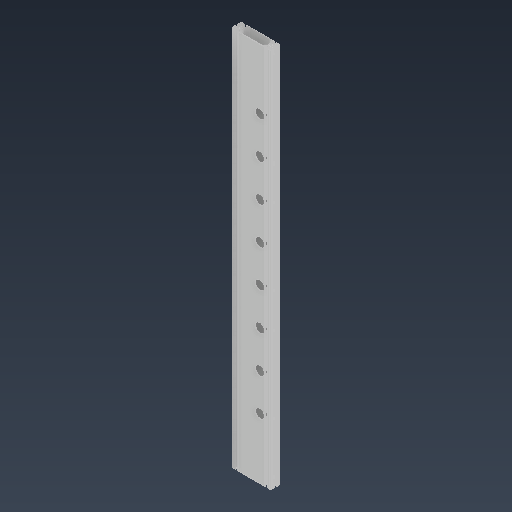
# Autodesk Inventor part: tallBeamLong
Saved by Autodesk Inventor 2021.4 (Build 254397000, 397)
## iProperties
Created: 2021-11-23
Part Number: tallBeamLong
Material: Generic
Document SubType Name: Modeling
Designer: jo_ki
Density: 1 g/cm^3
Appearance: Aluminum - Dark
Author: jo_ki
Autodesk Inventor part; units mm, degrees
ref_plane "YZ Plane" through (0, 0, 0) normal (1, 0, 0) x (0, 1, 0)
ref_plane "XZ Plane" through (0, 0, 0) normal (0, 1, 0) x (-1, 0, 0)
ref_plane "XY Plane" through (0, 0, 0) normal (0, 0, 1) x (1, 0, 0)
derived "Item_Profil_Hoch.ipt"
sketch "Skizze4" plane through (-54.5, 30, -20) normal (0, 1, 0) x (1, 0, 0)
  circle A0 centre (-5.5, -20) radius 3.4
  point P0 (54.5, -20)
sketch "Sketch9" plane through (0, 0, 0) normal (0, 1, 0) x (-1, 0, 0)
  line L0 (-78.3725, 16) -> (-78.3725, 12.3)
  arc A0 (-78.3725, 12.3) -> (-77.8725, 11.8) centre (-77.8725, 12.3) ccw
  line L1 (-77.8725, 11.8) -> (-72.4725, 11.8)
  arc A1 (-72.4725, 11.8) -> (-71.9725, 12.3) centre (-72.4725, 12.3) ccw
  line L2 (-71.9725, 12.3) -> (-71.9725, 17.7)
  arc A2 (-71.9725, 17.7) -> (-72.4725, 18.2) centre (-72.4725, 17.7) ccw
  line L3 (-72.4725, 18.2) -> (-76.1725, 18.2)
  arc A3 (-76.1725, 18.2) -> (-78.3725, 16) centre (-76.1725, 16) ccw
  line L4 (78.3725, -16) -> (78.3725, -12.3)
  arc A4 (78.3725, -12.3) -> (77.8725, -11.8) centre (77.8725, -12.3) ccw
  line L5 (77.8725, -11.8) -> (72.4725, -11.8)
  arc A5 (72.4725, -11.8) -> (71.9725, -12.3) centre (72.4725, -12.3) ccw
  line L6 (71.9725, -12.3) -> (71.9725, -17.7)
  arc A6 (71.9725, -17.7) -> (72.4725, -18.2) centre (72.4725, -17.7) ccw
  line L7 (72.4725, -18.2) -> (76.1725, -18.2)
  arc A7 (76.1725, -18.2) -> (78.3725, -16) centre (76.1725, -16) ccw
  line L8 (-76, -18.3725) -> (-72.3, -18.3725)
  arc A8 (-72.3, -18.3725) -> (-71.8, -17.8725) centre (-72.3, -17.8725) ccw
  line L9 (-71.8, -17.8725) -> (-71.8, -12.4725)
  arc A9 (-71.8, -12.4725) -> (-72.3, -11.9725) centre (-72.3, -12.4725) ccw
  line L10 (-72.3, -11.9725) -> (-77.7, -11.9725)
  arc A10 (-77.7, -11.9725) -> (-78.2, -12.4725) centre (-77.7, -12.4725) ccw
  line L11 (-78.2, -12.4725) -> (-78.2, -16.1725)
  arc A11 (-78.2, -16.1725) -> (-76, -18.3725) centre (-76, -16.1725) ccw
  line L12 (76, 18.3725) -> (72.3, 18.3725)
  arc A12 (72.3, 18.3725) -> (71.8, 17.8725) centre (72.3, 17.8725) ccw
  line L13 (71.8, 17.8725) -> (71.8, 12.4725)
  arc A13 (71.8, 12.4725) -> (72.3, 11.9725) centre (72.3, 12.4725) ccw
  line L14 (72.3, 11.9725) -> (77.7, 11.9725)
  arc A14 (77.7, 11.9725) -> (78.2, 12.4725) centre (77.7, 12.4725) ccw
  line L15 (78.2, 12.4725) -> (78.2, 16.1725)
  arc A15 (78.2, 16.1725) -> (76, 18.3725) centre (76, 16.1725) ccw
  circle A16 centre (60, 0) radius 3.4
  circle A17 centre (-60, 0) radius 3.4
  arc A18 (80, -5.5) -> (78.5, -4) centre (78.5, -5.5) ccw
  line L16 (80, -16) -> (80, -5.5)
  arc A19 (76, -20) -> (80, -16) centre (76, -16) ccw
  line L17 (65.5, -20) -> (76, -20)
  arc A20 (64, -18.5) -> (65.5, -20) centre (65.5, -18.5) ccw
  line L18 (64, -18.5) -> (64, -16.5)
  arc A21 (65, -15.5) -> (64, -16.5) centre (65, -16.5) ccw
  line L19 (65, -15.5) -> (66.5, -15.5)
  arc A22 (67, -16) -> (66.5, -15.5) centre (66.5, -16) ccw
  line L20 (67, -16) -> (67, -17.55)
  arc A23 (67, -17.55) -> (67.45, -18) centre (67.45, -17.55) ccw
  line L21 (67.45, -18) -> (67.5, -18)
  arc A24 (67.5, -18) -> (70, -15.5) centre (67.5, -15.5) ccw
  line L22 (70, -15.5) -> (70, -14.1924)
  arc A25 (70, -14.1924) -> (68.5355, -10.6569) centre (65, -14.1924) ccw
  line L23 (68.5355, -10.6569) -> (67.0931, -9.2145)
  arc A26 (67.0931, -9.2145) -> (63.5576, -7.75) centre (63.5576, -12.75) ccw
  line L24 (63.5576, -7.75) -> (56.4424, -7.75)
  arc A27 (56.4424, -7.75) -> (52.9069, -9.2145) centre (56.4424, -12.75) ccw
  line L25 (52.9069, -9.2145) -> (51.4645, -10.6569)
  arc A28 (51.4645, -10.6569) -> (50, -14.1924) centre (55, -14.1924) ccw
  line L26 (50, -14.1924) -> (50, -15.5)
  arc A29 (50, -15.5) -> (52.5, -18) centre (52.5, -15.5) ccw
  line L27 (52.5, -18) -> (52.55, -18)
  arc A30 (52.55, -18) -> (53, -17.55) centre (52.55, -17.55) ccw
  line L28 (53, -17.55) -> (53, -16)
  arc A31 (53.5, -15.5) -> (53, -16) centre (53.5, -16) ccw
  line L29 (53.5, -15.5) -> (55, -15.5)
  arc A32 (56, -16.5) -> (55, -15.5) centre (55, -16.5) ccw
  line L30 (56, -16.5) -> (56, -18.5)
  arc A33 (54.5, -20) -> (56, -18.5) centre (54.5, -18.5) ccw
  line L31 (-54.5, -20) -> (54.5, -20)
  arc A34 (-56, -18.5) -> (-54.5, -20) centre (-54.5, -18.5) ccw
  line L32 (-56, -18.5) -> (-56, -16.5)
  arc A35 (-55, -15.5) -> (-56, -16.5) centre (-55, -16.5) ccw
  line L33 (-55, -15.5) -> (-53.5, -15.5)
  arc A36 (-53, -16) -> (-53.5, -15.5) centre (-53.5, -16) ccw
  line L34 (-53, -16) -> (-53, -17.55)
  arc A37 (-53, -17.55) -> (-52.55, -18) centre (-52.55, -17.55) ccw
  line L35 (-52.55, -18) -> (-52.5, -18)
  arc A38 (-52.5, -18) -> (-50, -15.5) centre (-52.5, -15.5) ccw
  line L36 (-50, -15.5) -> (-50, -14.1924)
  arc A39 (-50, -14.1924) -> (-51.4645, -10.6569) centre (-55, -14.1924) ccw
  line L37 (-51.4645, -10.6569) -> (-52.9069, -9.2145)
  arc A40 (-52.9069, -9.2145) -> (-56.4424, -7.75) centre (-56.4424, -12.75) ccw
  line L38 (-56.4424, -7.75) -> (-63.5576, -7.75)
  arc A41 (-63.5576, -7.75) -> (-67.0931, -9.2145) centre (-63.5576, -12.75) ccw
  line L39 (-67.0931, -9.2145) -> (-68.5355, -10.6569)
  arc A42 (-68.5355, -10.6569) -> (-70, -14.1924) centre (-65, -14.1924) ccw
  line L40 (-70, -14.1924) -> (-70, -15.5)
  arc A43 (-70, -15.5) -> (-67.5, -18) centre (-67.5, -15.5) ccw
  line L41 (-67.5, -18) -> (-67.45, -18)
  arc A44 (-67.45, -18) -> (-67, -17.55) centre (-67.45, -17.55) ccw
  line L42 (-67, -17.55) -> (-67, -16)
  arc A45 (-66.5, -15.5) -> (-67, -16) centre (-66.5, -16) ccw
  line L43 (-66.5, -15.5) -> (-65, -15.5)
  arc A46 (-64, -16.5) -> (-65, -15.5) centre (-65, -16.5) ccw
  line L44 (-64, -16.5) -> (-64, -18.5)
  arc A47 (-65.5, -20) -> (-64, -18.5) centre (-65.5, -18.5) ccw
  line L45 (-76, -20) -> (-65.5, -20)
  arc A48 (-80, -16) -> (-76, -20) centre (-76, -16) ccw
  line L46 (-80, -5.5) -> (-80, -16)
  arc A49 (-78.5, -4) -> (-80, -5.5) centre (-78.5, -5.5) ccw
  line L47 (-78.5, -4) -> (-76.5, -4)
  arc A50 (-75.5, -5) -> (-76.5, -4) centre (-76.5, -5) ccw
  line L48 (-75.5, -5) -> (-75.5, -6.5)
  arc A51 (-76, -7) -> (-75.5, -6.5) centre (-76, -6.5) ccw
  line L49 (-76, -7) -> (-77.55, -7)
  arc A52 (-77.55, -7) -> (-78, -7.45) centre (-77.55, -7.45) ccw
  line L50 (-78, -7.45) -> (-78, -7.5)
  arc A53 (-78, -7.5) -> (-75.5, -10) centre (-75.5, -7.5) ccw
  line L51 (-75.5, -10) -> (-74.1924, -10)
  arc A54 (-74.1924, -10) -> (-70.6569, -8.5355) centre (-74.1924, -5) ccw
  line L52 (-70.6569, -8.5355) -> (-69.2145, -7.0931)
  arc A55 (-69.2145, -7.0931) -> (-67.75, -3.5576) centre (-72.75, -3.5576) ccw
  line L53 (-67.75, -3.5576) -> (-67.75, 3.5576)
  arc A56 (-67.75, 3.5576) -> (-69.2145, 7.0931) centre (-72.75, 3.5576) ccw
  line L54 (-69.2145, 7.0931) -> (-70.6569, 8.5355)
  arc A57 (-70.6569, 8.5355) -> (-74.1924, 10) centre (-74.1924, 5) ccw
  line L55 (-74.1924, 10) -> (-75.5, 10)
  arc A58 (-75.5, 10) -> (-78, 7.5) centre (-75.5, 7.5) ccw
  line L56 (-78, 7.5) -> (-78, 7.45)
  arc A59 (-78, 7.45) -> (-77.55, 7) centre (-77.55, 7.45) ccw
  line L57 (-77.55, 7) -> (-76, 7)
  arc A60 (-75.5, 6.5) -> (-76, 7) centre (-76, 6.5) ccw
  line L58 (-75.5, 6.5) -> (-75.5, 5)
  arc A61 (-76.5, 4) -> (-75.5, 5) centre (-76.5, 5) ccw
  line L59 (-76.5, 4) -> (-78.5, 4)
  arc A62 (-80, 5.5) -> (-78.5, 4) centre (-78.5, 5.5) ccw
  line L60 (-80, 16) -> (-80, 5.5)
  arc A63 (-76, 20) -> (-80, 16) centre (-76, 16) ccw
  line L61 (-65.5, 20) -> (-76, 20)
  arc A64 (-64, 18.5) -> (-65.5, 20) centre (-65.5, 18.5) ccw
  line L62 (-64, 18.5) -> (-64, 16.5)
  arc A65 (-65, 15.5) -> (-64, 16.5) centre (-65, 16.5) ccw
  line L63 (-65, 15.5) -> (-66.5, 15.5)
  arc A66 (-67, 16) -> (-66.5, 15.5) centre (-66.5, 16) ccw
  line L64 (-67, 16) -> (-67, 17.55)
  arc A67 (-67, 17.55) -> (-67.45, 18) centre (-67.45, 17.55) ccw
  line L65 (-67.45, 18) -> (-67.5, 18)
  arc A68 (-67.5, 18) -> (-70, 15.5) centre (-67.5, 15.5) ccw
  line L66 (-70, 15.5) -> (-70, 14.1924)
  arc A69 (-70, 14.1924) -> (-68.5355, 10.6569) centre (-65, 14.1924) ccw
  line L67 (-68.5355, 10.6569) -> (-67.0931, 9.2145)
  arc A70 (-67.0931, 9.2145) -> (-63.5576, 7.75) centre (-63.5576, 12.75) ccw
  line L68 (-63.5576, 7.75) -> (-56.4424, 7.75)
  arc A71 (-56.4424, 7.75) -> (-52.9069, 9.2145) centre (-56.4424, 12.75) ccw
  line L69 (-52.9069, 9.2145) -> (-51.4645, 10.6569)
  arc A72 (-51.4645, 10.6569) -> (-50, 14.1924) centre (-55, 14.1924) ccw
  line L70 (-50, 14.1924) -> (-50, 15.5)
  arc A73 (-50, 15.5) -> (-52.5, 18) centre (-52.5, 15.5) ccw
  line L71 (-52.5, 18) -> (-52.55, 18)
  arc A74 (-52.55, 18) -> (-53, 17.55) centre (-52.55, 17.55) ccw
  line L72 (-53, 17.55) -> (-53, 16)
  arc A75 (-53.5, 15.5) -> (-53, 16) centre (-53.5, 16) ccw
  line L73 (-53.5, 15.5) -> (-55, 15.5)
  arc A76 (-56, 16.5) -> (-55, 15.5) centre (-55, 16.5) ccw
  line L74 (-56, 16.5) -> (-56, 18.5)
  arc A77 (-54.5, 20) -> (-56, 18.5) centre (-54.5, 18.5) ccw
  line L75 (54.5, 20) -> (-54.5, 20)
  arc A78 (56, 18.5) -> (54.5, 20) centre (54.5, 18.5) ccw
  line L76 (56, 18.5) -> (56, 16.5)
  arc A79 (55, 15.5) -> (56, 16.5) centre (55, 16.5) ccw
  line L77 (55, 15.5) -> (53.5, 15.5)
  arc A80 (53, 16) -> (53.5, 15.5) centre (53.5, 16) ccw
  line L78 (53, 16) -> (53, 17.55)
  arc A81 (53, 17.55) -> (52.55, 18) centre (52.55, 17.55) ccw
  line L79 (52.55, 18) -> (52.5, 18)
  arc A82 (52.5, 18) -> (50, 15.5) centre (52.5, 15.5) ccw
  line L80 (50, 15.5) -> (50, 14.1924)
  arc A83 (50, 14.1924) -> (51.4645, 10.6569) centre (55, 14.1924) ccw
  line L81 (51.4645, 10.6569) -> (52.9069, 9.2145)
  arc A84 (52.9069, 9.2145) -> (56.4424, 7.75) centre (56.4424, 12.75) ccw
  line L82 (56.4424, 7.75) -> (63.5576, 7.75)
  arc A85 (63.5576, 7.75) -> (67.0931, 9.2145) centre (63.5576, 12.75) ccw
  line L83 (67.0931, 9.2145) -> (68.5355, 10.6569)
  arc A86 (68.5355, 10.6569) -> (70, 14.1924) centre (65, 14.1924) ccw
  line L84 (70, 14.1924) -> (70, 15.5)
  arc A87 (70, 15.5) -> (67.5, 18) centre (67.5, 15.5) ccw
  line L85 (67.5, 18) -> (67.45, 18)
  arc A88 (67.45, 18) -> (67, 17.55) centre (67.45, 17.55) ccw
  line L86 (67, 17.55) -> (67, 16)
  arc A89 (66.5, 15.5) -> (67, 16) centre (66.5, 16) ccw
  line L87 (66.5, 15.5) -> (65, 15.5)
  arc A90 (64, 16.5) -> (65, 15.5) centre (65, 16.5) ccw
  line L88 (64, 16.5) -> (64, 18.5)
  arc A91 (65.5, 20) -> (64, 18.5) centre (65.5, 18.5) ccw
  line L89 (76, 20) -> (65.5, 20)
  arc A92 (80, 16) -> (76, 20) centre (76, 16) ccw
  line L90 (80, 5.5) -> (80, 16)
  arc A93 (78.5, 4) -> (80, 5.5) centre (78.5, 5.5) ccw
  line L91 (78.5, 4) -> (76.5, 4)
  arc A94 (75.5, 5) -> (76.5, 4) centre (76.5, 5) ccw
  line L92 (75.5, 5) -> (75.5, 6.5)
  arc A95 (76, 7) -> (75.5, 6.5) centre (76, 6.5) ccw
  line L93 (76, 7) -> (77.55, 7)
  arc A96 (77.55, 7) -> (78, 7.45) centre (77.55, 7.45) ccw
  line L94 (78, 7.45) -> (78, 7.5)
  arc A97 (78, 7.5) -> (75.5, 10) centre (75.5, 7.5) ccw
  line L95 (75.5, 10) -> (74.1924, 10)
  arc A98 (74.1924, 10) -> (70.6569, 8.5355) centre (74.1924, 5) ccw
  line L96 (70.6569, 8.5355) -> (69.2145, 7.0931)
  arc A99 (69.2145, 7.0931) -> (67.75, 3.5576) centre (72.75, 3.5576) ccw
  line L97 (67.75, 3.5576) -> (67.75, -3.5576)
  arc A100 (67.75, -3.5576) -> (69.2145, -7.0931) centre (72.75, -3.5576) ccw
  line L98 (69.2145, -7.0931) -> (70.6569, -8.5355)
  arc A101 (70.6569, -8.5355) -> (74.1924, -10) centre (74.1924, -5) ccw
  line L99 (74.1924, -10) -> (75.5, -10)
  arc A102 (75.5, -10) -> (78, -7.5) centre (75.5, -7.5) ccw
  line L100 (78, -7.5) -> (78, -7.45)
  arc A103 (78, -7.45) -> (77.55, -7) centre (77.55, -7.45) ccw
  line L101 (77.55, -7) -> (76, -7)
  arc A104 (75.5, -6.5) -> (76, -7) centre (76, -6.5) ccw
  line L102 (75.5, -6.5) -> (75.5, -5)
  arc A105 (76.5, -4) -> (75.5, -5) centre (76.5, -5) ccw
  line L103 (76.5, -4) -> (78.5, -4)
  line L104 (-44.5, -17) -> (44.5, -17)
  arc A106 (44.5, -17) -> (47, -14.5) centre (44.5, -14.5) ccw
  line L105 (47, -14.5) -> (47, -12.8211)
  arc A107 (48.4645, -9.2855) -> (47, -12.8211) centre (52, -12.8211) ccw
  line L106 (48.4645, -9.2855) -> (51.05, -6.7)
  arc A108 (51.05, -6.7) -> (52.25, -4.5646) centre (49.75, -4.5646) ccw
  line L107 (52.25, -4.5646) -> (52.25, 4.5646)
  arc A109 (52.25, 4.5646) -> (51.05, 6.7) centre (49.75, 4.5646) ccw
  line L108 (51.05, 6.7) -> (48.4645, 9.2855)
  arc A110 (47, 12.8211) -> (48.4645, 9.2855) centre (52, 12.8211) ccw
  line L109 (47, 12.8211) -> (47, 14.5)
  arc A111 (47, 14.5) -> (44.5, 17) centre (44.5, 14.5) ccw
  line L110 (44.5, 17) -> (-44.5, 17)
  arc A112 (-44.5, 17) -> (-47, 14.5) centre (-44.5, 14.5) ccw
  line L111 (-47, 14.5) -> (-47, 12.8211)
  arc A113 (-48.4645, 9.2855) -> (-47, 12.8211) centre (-52, 12.8211) ccw
  line L112 (-48.4645, 9.2855) -> (-51.05, 6.7)
  arc A114 (-51.05, 6.7) -> (-52.25, 4.5646) centre (-49.75, 4.5646) ccw
  line L113 (-52.25, 4.5646) -> (-52.25, -4.5646)
  arc A115 (-52.25, -4.5646) -> (-51.05, -6.7) centre (-49.75, -4.5646) ccw
  line L114 (-51.05, -6.7) -> (-48.4645, -9.2855)
  arc A116 (-47, -12.8211) -> (-48.4645, -9.2855) centre (-52, -12.8211) ccw
  line L115 (-47, -12.8211) -> (-47, -14.5)
  arc A117 (-47, -14.5) -> (-44.5, -17) centre (-44.5, -14.5) ccw
  point P0 (0, 0)
  point P1 (0, 0)
derived "Mastersketch.ipt"
extrude "Extrusion1" add sketch "Sketch9" along normal mid plane 1540
sketch "Sketch3" plane through (0, 0, 0) normal (0, 0, 1) x (1, 0, 0)
  line L0 (80, -770) -> (80, 770) projected
  line L1 (-92.08, 0) -> (108.68, 0) projected
  point P0 (0, 0)
  point P1 (35, 525)
  dimension "d8" = 45
  dimension "d9" = 525
  measures "d8" distance from line of point (35, 525) L0
  measures "d9" distance from line of L1 point (35, 525)
hole "Hole1" at (35, 525, 0) direction (0, 0, -1) diameter 36 end through all both
pattern_linear "Rectangular Pattern1" count 8 spacing 150 along (0, -1, 0) of "Hole1"
equation "\"d2\" = feet_lengthCenter + profile_width"
equation "\"d8\" = handle_offsetTop"
equation "\"d10\" = handleHole_diameter"
equation "\"d27\" = handle_distance"
equation "\"feet_lengthCenter\" = 1500"
equation "\"profile_width\" = 40"
equation "\"handleHole_diameter\" = 36"
equation "\"handle_distance\" = 150"
equation "\"handle_offsetTop\" = 45"
body "Solid1"
